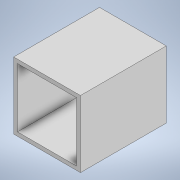
# Autodesk Inventor part: C_358_40_2
Saved by Autodesk Inventor 2020 (Build 240168000, 168)
## iProperties
Created: 2022-03-28
Part Number: C_358_40_2
Material: Genérico
Document SubType Name: Modeling
Designer: aarco
Density: 1 g/cm^3
Appearance: Valor por defecto
Author: aarco
Autodesk Inventor part; units mm, degrees
ref_plane "YZ Plane" through (0, 0, 0) normal (1, 0, 0) x (0, 1, 0)
ref_plane "XZ Plane" through (0, 0, 0) normal (0, 1, 0) x (-1, 0, 0)
ref_plane "XY Plane" through (0, 0, 0) normal (0, 0, 1) x (1, 0, 0)
sketch "Boceto1" plane through (0, 0, 0) normal (0, 0, 1) x (1, 0, 0)
  line L0 (-17.5, 17.5) -> (17.5, 17.5)
  line L1 (17.5, 17.5) -> (17.5, -17.5)
  line L2 (17.5, -17.5) -> (-17.5, -17.5)
  line L3 (-17.5, -17.5) -> (-17.5, 17.5)
  line L4 (-17.5, 17.5) -> (17.5, -17.5) construction
  line L5 (-15.5, 15.5) -> (15.5, 15.5)
  line L6 (15.5, 15.5) -> (15.5, -15.5)
  line L7 (15.5, -15.5) -> (-15.5, -15.5)
  line L8 (-15.5, -15.5) -> (-15.5, 15.5)
  line L9 (-15.5, 0) -> (-17.5, 0) construction
  line L10 (0, 15.5) -> (0, 17.5) construction
  line L11 (15.5, 0) -> (17.5, 0) construction
  line L12 (0, -15.5) -> (0, -17.5) construction
  point P0 (0, 0)
  point P1 (0, 0)
  dimension "d0" = 35
  dimension "d1" = 2
  constraints: 26 end point, 9 midpoint, 6 perpendicular, 4 parallel, 2 horizontal, 2 point on line, 1 coincident
  measures "d0" distance of L2.end L0.start
  measures "d1" distance of L10.start L10.end
extrude "Extrusión1" add sketch "Boceto1" along normal blind 45
